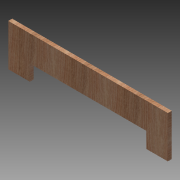
# Autodesk Inventor part: Chassis_Bumpermount_woodpiece
Saved by Autodesk Inventor 2014 (Build 180170000, 170)
## iProperties
Created: 2016-01-26
Part Number: Chassis_Bumpermount_woodpiece
Material: Generic
Document SubType Name: Modeling
Designer: shawnsargent
Density: 1 g/cm^3
Appearance: Birch - Natural Polished
Author: shawnsargent
Autodesk Inventor part; units mm, degrees
ref_plane "YZ Plane" through (0, 0, 0) normal (1, 0, 0) x (0, 1, 0)
ref_plane "XZ Plane" through (0, 0, 0) normal (0, 1, 0) x (-1, 0, 0)
ref_plane "XY Plane" through (0, 0, 0) normal (0, 0, 1) x (1, 0, 0)
sketch "Sketch1" plane through (0, 0, 0) normal (0, 0, 1) x (1, 0, 0)
  line L0 (178.5337, 8.656) -> (283.3087, 8.656)
  line L1 (283.3087, 8.656) -> (283.3087, -194.544)
  line L2 (283.3087, -194.544) -> (178.5337, -194.544)
  line L3 (178.5337, -194.544) -> (178.5337, 8.656)
  line L4 (178.5337, 8.656) -> (953.2337, 8.656)
  line L5 (953.2337, 8.656) -> (953.2337, -118.344)
  line L6 (953.2337, -118.344) -> (178.5337, -118.344)
  line L7 (178.5337, -118.344) -> (178.5337, 8.656)
  line L8 (953.2337, 8.656) -> (848.4587, 8.656)
  line L9 (848.4587, 8.656) -> (848.4587, -194.544)
  line L10 (848.4587, -194.544) -> (953.2337, -194.544)
  line L11 (953.2337, -194.544) -> (953.2337, 8.656)
  dimension "d21" = 104.775
  dimension "d22" = 203.2
  dimension "d23" = 774.7
  dimension "d24" = 127
  dimension "d25" = 104.775
  constraints: 24 end point, 6 parallel, 3 horizontal, 3 perpendicular
  measures "d21" distance of L1.end L2.end
  measures "d22" distance of L0.end L1.end
  measures "d23" distance of L5.end L6.end
  measures "d24" distance of L4.end L5.end
  measures "d25" distance of L10.end L9.end
extrude "Extrusion3" add sketch "Sketch1" along normal blind 19.05
body "Solid2"
